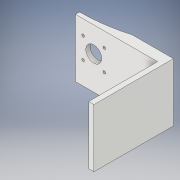
# Autodesk Inventor part: CA002
Saved by Autodesk Inventor 2017 SP1 (Build 210196100, 196)
## iProperties
Created: 2017-07-18
Part Number: CA002
Material: ABS Plastic
Document SubType Name: Modeling
Designer: zallen
Density: 1.06 g/cm^3
Appearance: CR White
Author: zallen
Autodesk Inventor part; units mm, degrees
ref_plane "YZ Plane" through (0, 0, 0) normal (1, 0, 0) x (0, 1, 0)
ref_plane "XZ Plane" through (0, 0, 0) normal (0, 1, 0) x (-1, 0, 0)
ref_plane "XY Plane" through (0, 0, 0) normal (0, 0, 1) x (1, 0, 0)
sketch "Sketch1" plane through (0, 0, 0) normal (0, 0, 1) x (1, 0, 0)
  line L0 (0, 0) -> (330, 0)
  line L1 (330, 0) -> (330, 510)
  line L2 (330, 510) -> (0, 510)
  line L3 (0, 510) -> (0, 0)
  dimension "d0" = 330
  dimension "d1" = 510
  constraints: 8 end point, 2 parallel, 1 horizontal, 1 perpendicular
  measures "d0" distance of L2.end L1.end
  measures "d1" distance of L1.end L0.end
extrude "Extrusion1" add sketch "Sketch1" along normal blind 150
sketch "Sketch2" plane through (0, 0, 0) normal (0, -1, 0) x (1, 0, 0)
  circle A0 centre (165, -304.672) radius 315
  line L0 (85, 0) -> (245, 0)
  line L1 (0, 0) -> (330, 0) projected
  circle A1 centre (165, -304.672) radius 317
  point P0 (165, 0)
  point P1 (165, 0)
  dimension "d4" = 630
  dimension "d8" = 160
  dimension "d9" = 2
  constraints: 2 centre point, 2 end point, 2 midpoint, 2 point on circle, 2 point on line, 1 coincident, 1 vertical alignment
  measures "d4" diameter of A0
  measures "d8" distance of L0.start L0.end
  measures "d9" radial gap between concentric circles of A0 A1
extrude "Extrusion2" cut sketch "Sketch2" against normal through all
sketch "Sketch3" plane through (0, 0, 150) normal (0, 0, 1) x (1, 0, 0)
  line L0 (0, 0) -> (330, 0) projected
  line L1 (330, 0) -> (330, 510) projected
  line L2 (330, 510) -> (0, 510) projected
  line L3 (0, 510) -> (0, 0) projected
  line L4 (10, 10) -> (320, 10)
  line L5 (320, 10) -> (320, 500)
  line L6 (320, 500) -> (10, 500)
  line L7 (10, 500) -> (10, 10)
  dimension "d10" = 10
  constraints: 8 end point, 3 other
  measures "d10" distance between parallel lines of L3 L7
extrude "Extrusion3" cut sketch "Sketch3" against normal blind 130 contours L7 L6 L5 L4
sketch "Sketch4" plane through (0, 0, 20) normal (0, 0, 1) x (1, 0, 0)
  line L0 (10, 500) -> (320, 500) construction
  line L1 (85, 500) -> (245, 500) construction
  line L2 (245, 500) -> (245, 10) construction
  line L3 (245, 10) -> (85, 10) construction
  line L4 (85, 10) -> (85, 500) construction
  line L5 (320, 10) -> (10, 10) construction
  line L6 (85, 500) -> (245, 500) construction
  line L7 (245, 500) -> (245, 455) construction
  line L8 (245, 455) -> (85, 455) construction
  line L9 (85, 455) -> (85, 500) construction
  line L10 (85, 455) -> (245, 455) construction
  line L11 (245, 455) -> (245, 400) construction
  line L12 (245, 400) -> (85, 400) construction
  line L13 (85, 400) -> (85, 455) construction
  line L14 (85, 400) -> (245, 400) construction
  line L15 (245, 400) -> (245, 345) construction
  line L16 (245, 345) -> (85, 345) construction
  line L17 (85, 345) -> (85, 400) construction
  line L18 (85, 345) -> (245, 345) construction
  line L19 (245, 345) -> (245, 290) construction
  line L20 (245, 290) -> (85, 290) construction
  line L21 (85, 290) -> (85, 345) construction
  line L22 (85, 290) -> (245, 290) construction
  line L23 (245, 290) -> (245, 235) construction
  line L24 (245, 235) -> (85, 235) construction
  line L25 (85, 235) -> (85, 290) construction
  circle A0 centre (130.3559, 262.5) radius 15
  circle A1 centre (199.6441, 262.5) radius 15
  line L26 (130.3559, 262.5) -> (199.6441, 262.5) construction
  point P0 (0, 0)
  point P1 (165, 500)
  point P2 (165, 500)
  point P3 (165, 262.5)
  point P4 (165, 235)
  point P5 (245, 262.5)
  dimension "d13" = 160
  dimension "d14" = 45
  dimension "d15" = 55
  dimension "d16" = 55
  dimension "d17" = 55
  dimension "d18" = 55
  dimension "d19" = 30
  dimension "d20" = 30
  dimension "d21" = 69.2883
  constraints: 50 end point, 12 parallel, 7 horizontal, 7 point on line, 6 perpendicular, 5 midpoint, 2 centre point, 1 coincident, 1 horizontal alignment, 1 vertical alignment
  measures "d13" distance of L2.end L3.end
  measures "d14" distance of L6.end L7.end
  measures "d15" distance of L10.end L11.end
  measures "d16" distance of L14.end L15.end
  measures "d17" distance of L18.end L19.end
  measures "d18" distance of L22.end L23.end
  measures "d19" diameter of A0
  measures "d20" diameter of A1
  measures "d21" distance of L26.start L26.end
extrude "Extrusion4" cut sketch "Sketch4" against normal through all
sketch "Sketch5" plane through (0, 0, 150) normal (0, 0, 1) x (1, 0, 0)
  line L0 (330, 510) -> (0, 510) projected
  line L1 (330, 0) -> (330, 510) projected
  line L2 (0, 510) -> (330, 510)
  line L3 (330, 510) -> (330, 310)
  line L4 (330, 310) -> (0, 310)
  line L5 (0, 310) -> (0, 510)
  line L6 (0, 510) -> (0, 0) projected
  line L7 (330, 0) -> (0, 0)
  line L8 (0, 0) -> (0, 200)
  line L9 (0, 200) -> (330, 200)
  line L10 (330, 200) -> (330, 0)
  line L11 (0, 0) -> (330, 0) projected
  line L12 (330, 510) -> (165, 510)
  line L13 (165, 0) -> (330, 0)
  line L14 (330, 0) -> (330, 510)
  line L15 (0, 510) -> (165, 510)
  line L16 (165, 510) -> (165, 0)
  line L17 (165, 0) -> (0, 0)
  line L18 (0, 0) -> (0, 510)
  dimension "d24" = 200
  dimension "d25" = 200
  constraints: 30 end point, 7 parallel, 4 horizontal, 3 perpendicular, 2 point on line, 1 midpoint
  measures "d24" distance of L2.end L3.end
  measures "d25" distance of L7.end L8.end
extrude "Extrusion5" cut sketch "Sketch5" against normal through all contours L1 L4 L16 L0 | L16 L4 L5 L0 | L16 L9 L6 L4 | L1 L7 L16 L9 | L16 L7 L6 L9
sketch "Sketch6" plane through (0, 0, 20) normal (0, 0, 1) x (1, 0, 0)
  circle A0 centre (199.6441, 262.5) radius 15 construction
  line L0 (179.6441, 242.5) -> (219.6441, 242.5) construction
  line L1 (219.6441, 242.5) -> (219.6441, 282.5) construction
  line L2 (219.6441, 282.5) -> (179.6441, 282.5) construction
  line L3 (179.6441, 282.5) -> (179.6441, 242.5) construction
  circle A1 centre (219.6441, 282.5) radius 2.5
  circle A2 centre (219.6441, 242.5) radius 2.5
  circle A3 centre (179.6441, 242.5) radius 2.5
  circle A4 centre (179.6441, 282.5) radius 2.5
  point P0 (0, 0)
  point P1 (199.6441, 282.5)
  point P2 (219.6441, 262.5)
  dimension "d28" = 40
  dimension "d29" = 40
  dimension "d30" = 5
  dimension "d31" = 5
  dimension "d32" = 5
  dimension "d33" = 5
  constraints: 8 end point, 4 centre point, 4 coincident, 2 midpoint, 2 parallel, 1 horizontal, 1 horizontal alignment, 1 perpendicular, 1 vertical alignment
  measures "d28" distance of L2.end L1.end
  measures "d29" distance of L1.end L0.end
  measures "d30" diameter of A1
  measures "d31" diameter of A2
  measures "d32" diameter of A3
  measures "d33" diameter of A4
extrude "Extrusion6" cut sketch "Sketch6" against normal through all
body "Solid1"
